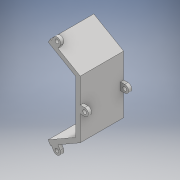
# Autodesk Inventor part: Capture Zone3
Saved by Autodesk Inventor 2018 (Build 220112000, 112)
## iProperties
Created: 2017-10-22
Part Number: Capture Zone3
Material: Generic
Document SubType Name: Modeling
Designer: BrisbaneMatt
Density: 1 g/cm^3
Appearance: Default
Author: BrisbaneMatt
Autodesk Inventor part; units mm, degrees
ref_plane "YZ Plane" through (0, 0, 0) normal (1, 0, 0) x (0, 1, 0)
ref_plane "XZ Plane" through (0, 0, 0) normal (0, 1, 0) x (-1, 0, 0)
ref_plane "XY Plane" through (0, 0, 0) normal (0, 0, 1) x (1, 0, 0)
sketch "Sketch1" plane through (0, 0, 0) normal (0, 1, 0) x (-1, 0, 0)
  line L0 (0, 0) -> (0, -48.498)
  line L1 (0, 0) -> (25.5001, 14.7225)
  line L2 (0, 0) -> (29.445, 0) construction
  line L3 (0, -48.498) -> (25.5001, -63.2205)
  line L4 (0, -48.498) -> (29.445, -48.498) construction
  line L5 (25.5001, -63.2205) -> (23.5001, -66.6846)
  line L6 (0, -46.9861) -> (-4, -46.9861)
  line L7 (-4, -46.9861) -> (-4, -50.8074)
  line L8 (-4, -50.8074) -> (23.5001, -66.6846)
  line L9 (1.1556, 0.6672) -> (-0.8444, 4.1313)
  line L10 (-0.8444, 4.1313) -> (-4, 2.3094)
  line L11 (-4, 2.3094) -> (-4, -46.9861)
  line L12 (-0.8444, 4.1313) -> (23.5001, 18.1866)
  line L13 (23.5001, 18.1866) -> (25.5001, 14.7225)
  dimension "d0" = 48.498
  dimension "d1" = 29.445
  dimension "d2" = 30
  dimension "d3" = 29.445
  dimension "d4" = 30
  dimension "d5" = 4
  dimension "d6" = 4
  dimension "d7" = 4
  constraints: 28 end point, 7 perpendicular, 4 point on line, 2 equal length, 2 horizontal, 1 collinear, 1 vertical
  measures "d0" distance of L0.start L0.end
  measures "d1" distance of L0.start L1.end
  measures "d2" angle of L2 L1
  measures "d3" distance of L0.end L3.end
  measures "d4" angle of L3 L4
  measures "d5" distance of L3.end L5.end
  measures "d6" distance of L6.start L6.end
  measures "d7" distance of L9.start L9.end
extrude "Extrusion1" add sketch "Sketch1" along normal blind 40
sketch "Sketch2" plane through (0, 0, 0) normal (0, -1, 0) x (1, 0, 0)
  line L0 (0, 0) -> (-25.5001, 14.7225) projected
  line L1 (-25.5001, 14.7225) -> (-23.1946, 18.7157)
  line L2 (-25.5001, 14.7225) -> (-23.5001, 18.1866) projected
  line L3 (-23.1946, 18.7157) -> (-25.5001, 14.7225)
  line L4 (-25.5001, 14.7225) -> (-21.5069, 12.417)
  line L5 (-21.5069, 12.417) -> (-17.5069, 19.3452)
  circle A0 centre (-17.5069, 19.3452) radius 1.75
  circle A1 centre (-17.5069, 19.3452) radius 3.5
  line L6 (-20.538, 21.0952) -> (-22.538, 17.6311)
  line L7 (-23.5001, 18.1866) -> (4, 2.3094) projected
  line L8 (-14.4758, 17.5952) -> (-16.4758, 14.1311)
  dimension "d10" = 4.611
  dimension "d11" = 4.611
  dimension "d12" = 8
  dimension "d13" = 3.5
  dimension "d14" = 7
  constraints: 12 end point, 2 centre point, 2 coincident, 2 collinear, 2 perpendicular, 2 point on circle, 1 parallel, 1 point on line, 1 tangent
  measures "d10" distance of L0.end L1.end
  measures "d11" distance of L0.end L4.end
  measures "d12" distance of L4.end L5.end
  measures "d13" diameter of A0
  measures "d14" diameter of A1
extrude "Extrusion2" add sketch "Sketch2" against normal blind 3 contours A1
sketch "Sketch3" plane through (-17.5069, 3, 19.3452) normal (0, 1, 0) x (1, 0, 0)
  circle A0 centre (0, 0) radius 1.75 projected
  line L0 (0, 0) -> (-2, 3.4641)
  line L1 (-5.9932, 1.1586) -> (21.5069, 17.0358) projected
  line L2 (-2, 3.4641) -> (-5.0311, 1.7141)
  line L3 (-5.0311, 1.7141) -> (-3.0311, -1.75)
  circle A1 centre (0, 0) radius 3.5 projected
  line L4 (-2, 3.4641) -> (1.0311, 5.2141)
  line L5 (1.0311, 5.2141) -> (2.9919, 1.8179)
  line L6 (2.9919, 1.8179) -> (1.5256, 0.9713)
  line L7 (1.5256, 0.9713) -> (0.9971, 2.6723)
  line L8 (0.9971, 2.6723) -> (-1.1427, 2.5009)
  line L9 (-1.1427, 2.5009) -> (-2.2108, 1.3125)
  line L10 (-2.2108, 1.3125) -> (-2.3481, -0.99)
  line L11 (-2.3481, -0.99) -> (-3.0311, -1.75)
  point P0 (17.5069, 19.3452)
  dimension "d17" = 3.5
  dimension "d18" = 3.5
  constraints: 22 end point, 4 perpendicular, 2 point on line, 1 parallel, 2 other
  measures "d17" distance of L0.end L2.end
  measures "d18" distance of L0.end L4.end
extrude "Extrusion3" add sketch "Sketch3" against normal blind 3 contours L9 L10 L11 A1 L0 | L0 A1 L6 L7 L8 L9 | A1 L3 L1 L0 | L0 L1 L5 A1
sketch "Sketch4" plane through (0, 0, 0) normal (0, -1, 0) x (1, 0, 0)
  line L0 (-23.5001, -66.6846) -> (-25.5001, -63.2205) projected
  line L1 (-23.5001, -66.6846) -> (-21.1946, -70.6778)
  line L2 (-21.1946, -70.6778) -> (-23.5001, -66.6846)
  line L3 (-25.5001, -63.2205) -> (0, -48.498) projected
  line L4 (-25.5001, -63.2205) -> (-21.5069, -60.915)
  line L5 (-21.5069, -60.915) -> (-17.5069, -67.8432)
  circle A0 centre (-17.5069, -67.8432) radius 1.75
  circle A1 centre (-17.5069, -67.8432) radius 3.5
  line L6 (-19.5069, -64.3791) -> (-22.538, -66.1291)
  line L7 (4, -50.8074) -> (-23.5001, -66.6846) projected
  line L8 (-22.538, -66.1291) -> (-20.538, -69.5932)
  line L9 (-19.5069, -64.3791) -> (-16.4758, -62.6291)
  line L10 (-16.4758, -62.6291) -> (-14.4758, -66.0932)
  point P0 (0, 0)
  dimension "d21" = 4.611
  dimension "d22" = 4.611
  dimension "d23" = 8
  dimension "d24" = 3.5
  dimension "d25" = 7
  dimension "d26" = 3.5
  dimension "d27" = 3.5
  constraints: 16 end point, 3 perpendicular, 3 point on line, 2 centre point, 2 coincident, 2 collinear, 2 point on circle, 1 midpoint
  measures "d21" distance of L0.start L1.end
  measures "d22" distance of L0.end L4.end
  measures "d23" distance of L4.end L5.end
  measures "d24" diameter of A0
  measures "d25" diameter of A1
  measures "d26" distance of L6.start L6.end
  measures "d27" distance of L6.start L9.end
extrude "Extrusion4" add sketch "Sketch4" against normal blind 3 contours L6 L5 A1 L8 | L7 L10 A1 L5 | A1
sketch "Sketch5" plane through (0, 0, 0) normal (0, -1, 0) x (1, 0, 0)
  line L0 (0, -48.498) -> (0, 0) projected
  line L1 (0, -24.249) -> (8, -24.249)
  circle A0 centre (8, -24.249) radius 1.75
  circle A1 centre (8, -24.249) radius 3.5
  line L2 (4, 2.3094) -> (4, -50.8074) projected
  line L3 (4, -24.249) -> (4, -27.749)
  line L4 (4, -27.749) -> (8, -27.749)
  line L5 (4, -24.249) -> (4, -20.749)
  line L6 (4, -20.749) -> (8, -20.749)
  dimension "d30" = 8
  dimension "d31" = 3.5
  dimension "d32" = 7
  constraints: 10 end point, 2 centre point, 2 coincident, 2 midpoint, 2 perpendicular, 2 point on circle, 2 point on line, 1 horizontal
  measures "d30" distance of L1.start L1.end
  measures "d31" diameter of A0
  measures "d32" diameter of A1
extrude "Extrusion5" add sketch "Sketch5" against normal blind 3
sketch "Sketch6" plane through (0, 40, 0) normal (0, 1, 0) x (1, 0, 0)
  line L0 (4, -2.3094) -> (4, 50.8074) projected
  line L1 (4, 24.249) -> (8, 24.249)
  circle A0 centre (8, 24.249) radius 1.75
  circle A1 centre (8, 24.249) radius 3.5
  line L2 (4, 27.749) -> (4, 50.8074) projected
  line L3 (4, 24.249) -> (4, 27.749)
  line L4 (8, 27.749) -> (4, 27.749) projected
  line L5 (4, 27.749) -> (8, 27.749)
  line L6 (4, 24.249) -> (4, 20.749)
  line L7 (4, 20.749) -> (8, 20.749) projected
  line L8 (4, 20.749) -> (8, 20.749)
  point P0 (0, 0)
  dimension "d35" = 4
  dimension "d36" = 3.5
  dimension "d37" = 7
  constraints: 10 end point, 2 centre point, 2 coincident, 1 collinear, 1 horizontal, 1 midpoint, 1 perpendicular, 1 point on line, 1 vertical
  measures "d35" distance of L1.start L1.end
  measures "d36" diameter of A0
  measures "d37" diameter of A1
extrude "Extrusion6" add sketch "Sketch6" against normal blind 3
body "Solid1"
